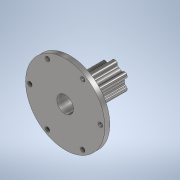
# Autodesk Inventor part: Rotor_Mount
Saved by Autodesk Inventor 2021 (Build 250183000, 183)
## iProperties
Created: 2021-03-26
Part Number: Rotor_Mount
Material: Stainless Steel
Document SubType Name: Modeling
Designer: lucia
Density: 8 g/cm^3
Appearance: Semi-Polished
Author: lucia
Autodesk Inventor part; units mm, degrees
ref_plane "YZ Plane" through (0, 0, 0) normal (1, 0, 0) x (0, 1, 0)
ref_plane "XZ Plane" through (0, 0, 0) normal (0, 1, 0) x (-1, 0, 0)
ref_plane "XY Plane" through (0, 0, 0) normal (0, 0, 1) x (1, 0, 0)
sketch "Sketch1" plane through (0, 0, 0) normal (0, 0, 1) x (1, 0, 0)
  circle A0 centre (0, 0) radius 39.624
  circle A1 centre (0, 0) radius 10.668
  dimension "d0" = 79.248
  dimension "d1" = 21.336
  constraints: 2 centre point, 2 coincident
  measures "d0" diameter of A0
  measures "d1" diameter of A1
extrude "Extrusion1" add sketch "Sketch1" along normal blind 12.7
sketch "Sketch2" plane through (0, 0, 0) normal (0, 0, -1) x (-1, 0, 0)
  circle A0 centre (0, 0) radius 39.624
  circle A1 centre (0, 0) radius 50.8
  line L0 (0, 0) -> (0, 50.8)
  circle A2 centre (0, 0) radius 39.624 projected
  line L1 (0, 0) -> (25.4, 43.9941)
  line L2 (-50.8, 0) -> (50.8, 0)
  line L3 (0, 0) -> (-25.4, 43.9941)
  line L4 (0, 0) -> (25.4, -43.9941)
  line L5 (0, 0) -> (-25.4, -43.9941)
  circle A3 centre (22.606, 39.1547) radius 2.7781
  circle A4 centre (45.212, 0) radius 2.7781
  circle A5 centre (-22.606, 39.1547) radius 2.7781
  circle A6 centre (-45.212, 0) radius 2.7781
  circle A7 centre (22.606, -39.1547) radius 2.7781
  circle A8 centre (-22.606, -39.1547) radius 2.7781
  dimension "d4" = 79.248
  dimension "d5" = 101.6
  dimension "d38" = 30
  dimension "d39" = 45.212
  dimension "d40" = 45.212
  dimension "d41" = 5.5563
  dimension "d42" = 5.5563
  constraints: 12 end point, 8 centre point, 7 symmetric about line, 4 point on circle, 2 coincident, 2 point on line, 1 midpoint, 1 perpendicular, 1 vertical, 4 other
  measures "d4" diameter of A0
  measures "d5" diameter of A1
  measures "d38" angle of L0 L1
  measures "d39" distance of point (0, 0) A3.centre
  measures "d40" distance of point (0, 0) A4.centre
  measures "d41" diameter of A4
  measures "d42" diameter of A3
extrude "Extrusion2" add sketch "Sketch2" against normal blind 12.7 contours L2 A4 A1 L4 A7 A0 | A0 L1 A3 A1 L2 A4 | A0 L0 A1 L1 A3 | L4 A7 A1 L5 A8 A0 | A4 L2 | L2 A4 | A0 L3 A5 A1 L0 | A3 L1 | L1 A3 | L5 A8 A1 L2 A6 A0 | A7 L4 | L4 A7 | L2 A6 A1 L3 A5 A0 | A8 L5 | L5 A8 | A6 L2 | L2 A6 | A5 L3 | L3 A5
sketch "Sketch3" plane through (0, 0, 0) normal (0, 0, -1) x (-1, 0, 0)
  circle A0 centre (0, 0) radius 10.668
  circle A1 centre (0, 0) radius 12.7
  dimension "d21" = 21.336
  dimension "d22" = 25.4
  constraints: 2 centre point, 2 coincident
  measures "d21" diameter of A0
  measures "d22" diameter of A1
extrude "Extrusion3" add sketch "Sketch3" along normal blind 50.8
sketch "Sketch4" plane through (0, 0, -50.8) normal (0, 0, -1) x (-1, 0, 0)
  circle A0 centre (0, 0) radius 12.7
  circle A1 centre (0, 0) radius 17.78
  line L0 (0, 0) -> (0, 17.78)
  line L1 (0, 0) -> (3.287, 12.2673)
  circle A2 centre (0, 0) radius 12.7 projected
  line L2 (0, 0) -> (-3.287, 12.2673)
  line L3 (3.287, 12.2673) -> (3.287, 17.4735)
  line L4 (-3.287, 12.2673) -> (-3.287, 17.4735)
  arc A3 (3.287, 14.082) -> (4.8558, 11.735) centre (5.827, 14.082) ccw
  arc A4 (3.287, 15.2217) -> (0.8715, 17.7586) centre (0.747, 15.2217) ccw
  arc A5 (-0.8715, 17.7586) -> (-3.287, 15.2217) centre (-0.747, 15.2217) ccw
  arc A6 (-4.8558, 11.735) -> (-3.287, 14.082) centre (-5.827, 14.082) ccw
  point P0 (-4.8558, 11.735)
  point P1 (4.8558, 11.735)
  dimension "d25" = 25.4
  dimension "d26" = 35.56
  dimension "d27" = 15
  dimension "d28" = 15
  dimension "d29" = 2.54
  dimension "d30" = 2.54
  dimension "d31" = 2.54
  dimension "d32" = 2.54
  constraints: 17 point on circle, 10 end point, 8 tangent, 6 centre point, 4 point on line, 2 coincident, 2 vertical, 1 parallel
  measures "d25" diameter of A0
  measures "d26" diameter of A1
  measures "d27" angle of L0 L1
  measures "d28" angle of L0 L2
  measures "d29" radius of A6
  measures "d30" radius of A5
  measures "d31" radius of A4
  measures "d32" radius of A3
extrude "Extrusion4" add sketch "Sketch4" against normal blind 38.1 contours A0 L3 A3 | A6 L4 A0 | A0 L0 A1 A4 L3 | L4 A5 A1 L0 A0
pattern_circular "Circular Pattern2" count 6 over 360 about axis through (0, 0, 0) along (0, 0, -1) of "Extrusion4"
sketch "Sketch5" plane through (0, 0, 0) normal (0, 0, -1) x (-1, 0, 0)
  circle A0 centre (0, 0) radius 39.624
  circle A1 centre (0, 0) radius 50.8
  line L0 (0, 0) -> (0, 50.8)
  circle A2 centre (0, 0) radius 39.624
  line L1 (0, 0) -> (25.4, 43.9941)
  line L2 (-50.8, 0) -> (50.8, 0)
  line L3 (0, 0) -> (-25.4, 43.9941)
  line L4 (0, 0) -> (25.4, -43.9941)
  line L5 (0, 0) -> (-25.4, -43.9941)
  circle A3 centre (22.606, 39.1547) radius 2.7781
  circle A4 centre (45.212, 0) radius 2.7781
  circle A5 centre (-22.606, 39.1547) radius 2.7781
  circle A6 centre (-45.212, 0) radius 2.7781
  circle A7 centre (22.606, -39.1547) radius 2.7781
  circle A8 centre (-22.606, -39.1547) radius 2.7781
  dimension "d43" = 79.248
  dimension "d44" = 101.6
  dimension "d45" = 30
  dimension "d46" = 45.212
  dimension "d47" = 45.212
  dimension "d48" = 5.5563
  dimension "d49" = 5.5563
  constraints: 12 end point, 9 centre point, 7 symmetric about line, 4 point on circle, 2 coincident, 2 point on line, 1 midpoint, 1 perpendicular, 1 vertical, 4 other
  measures "d43" diameter of A0
  measures "d44" diameter of A1
  measures "d45" angle of L0 L1
  measures "d46" distance of point (0, 0) A3.centre
  measures "d47" distance of point (0, 0) A4.centre
  measures "d48" diameter of A4
  measures "d49" diameter of A3
extrude "Extrusion5" cut sketch "Sketch5" against normal blind 6.35 contours L2 A4 A1 L4 A7 A0 | A0 L1 A3 A1 L2 A4 | A0 L0 A1 L1 A3 | L4 A7 A1 L5 A8 A0 | A4 L2 | L2 A4 | A0 L3 A5 A1 L0 | A3 L1 | L1 A3 | L5 A8 A1 L2 A6 A0 | A7 L4 | L4 A7 | L2 A6 A1 L3 A5 A0 | A8 L5 | L5 A8 | A6 L2 | L2 A6 | A5 L3 | L3 A5
sketch "Sketch6" plane through (0, 0, 6.35) normal (0, 0, -1) x (-1, 0, 0)
  circle A0 centre (0, 0) radius 39.624
  circle A1 centre (0, 0) radius 50.8
  line L0 (0, 0) -> (0, 50.8)
  circle A2 centre (0, 0) radius 39.624
  line L1 (0, 0) -> (25.4, 43.9941)
  line L2 (-50.8, 0) -> (50.8, 0)
  line L3 (0, 0) -> (-25.4, 43.9941)
  line L4 (0, 0) -> (25.4, -43.9941)
  line L5 (0, 0) -> (-25.4, -43.9941)
  circle A3 centre (22.606, 39.1547) radius 2.7781
  circle A4 centre (45.212, 0) radius 2.7781
  circle A5 centre (-22.606, 39.1547) radius 2.7781
  circle A6 centre (-45.212, 0) radius 2.7781
  circle A7 centre (22.606, -39.1547) radius 2.7781
  circle A8 centre (-22.606, -39.1547) radius 2.7781
  dimension "d53" = 79.248
  dimension "d54" = 101.6
  dimension "d55" = 30
  dimension "d56" = 45.212
  dimension "d57" = 45.212
  dimension "d58" = 5.5563
  dimension "d59" = 5.5563
  constraints: 12 end point, 9 centre point, 7 symmetric about line, 4 point on circle, 2 coincident, 2 point on line, 1 midpoint, 1 perpendicular, 1 vertical, 4 other
  measures "d53" diameter of A0
  measures "d54" diameter of A1
  measures "d55" angle of L0 L1
  measures "d56" distance of point (0, 0) A3.centre
  measures "d57" distance of point (0, 0) A4.centre
  measures "d58" diameter of A4
  measures "d59" diameter of A3
extrude "Extrusion6" cut sketch "Sketch6" against normal blind 6.35 contours A4 L2 | L2 A4 | A3 L1 | L1 A3 | A7 L4 | L4 A7 | A8 L5 | L5 A8 | A6 L2 | L2 A6 | A5 L3 | L3 A5
equation "\"d0\" = 19.812 * scale"
equation "\"d2\" = 3.175 * scale"
equation "\"d4\" = 19.812 * scale"
equation "\"d5\" = 25.4 * scale"
equation "\"d39\" = 11.303 * scale"
equation "\"d40\" = 11.303 * scale"
equation "\"d16\" = 3.175 * scale"
equation "\"d23\" = 12.7 * scale"
equation "\"d29\" = 0.635 * scale"
equation "\"d30\" = 0.635 * scale"
equation "\"d31\" = 0.635 * scale"
equation "\"d32\" = 0.635 * scale"
equation "\"d33\" = 9.525 * scale"
equation "\"d43\" = 19.812 * d50"
equation "\"d44\" = 25.4 * d50"
equation "\"d46\" = 11.303 * d50"
equation "\"d47\" = 11.303 * d50"
equation "\"d51\" = 1.5875 * scale"
equation "\"d53\" = 19.812 * d60"
equation "\"d54\" = 25.4 * d60"
equation "\"d56\" = 11.303 * d60"
equation "\"d57\" = 11.303 * d60"
equation "\"d61\" = 1.5875 * scale"
equation "\"radius\" = 3.175"
equation "\"scale\" = 4"
equation "\"d50\" = 4"
equation "\"d60\" = 4"
body "Solid1"
